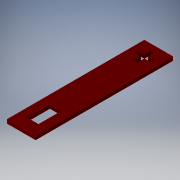
# Autodesk Inventor part: Brazo_Superior
Saved by Autodesk Inventor 2019 (Build 230136000, 136)
## iProperties
Created: 2020-02-09
Part Number: Brazo_Superior
Material: Generic
Document SubType Name: Modeling
Designer: Omar
Density: 1 g/cm^3
Appearance: Default
Author: Omar
Autodesk Inventor part; units mm, degrees
ref_plane "YZ Plane" through (0, 0, 0) normal (1, 0, 0) x (0, 1, 0)
ref_plane "XZ Plane" through (0, 0, 0) normal (0, 1, 0) x (-1, 0, 0)
ref_plane "XY Plane" through (0, 0, 0) normal (0, 0, 1) x (1, 0, 0)
sketch "Sketch1" plane through (0, 0, 0) normal (0, 1, 0) x (-1, 0, 0)
  line L0 (88.91, 20) -> (92.09, 20)
  line L1 (102.5, 9.09) -> (87.5, 9.09)
  line L2 (87.5, 9.09) -> (87.5, 5.91)
  line L3 (87.5, 5.91) -> (102.5, 5.91)
  line L4 (102.5, 5.91) -> (102.5, 9.09)
  line L5 (96.59, 15) -> (93.41, 15)
  line L6 (93.41, 15) -> (93.41, 0)
  line L7 (93.41, 0) -> (96.59, 0)
  line L8 (96.59, 0) -> (96.59, 15)
  line L9 (96.59, 15) -> (93.41, 0) construction
  line L10 (93.41, 15) -> (96.59, 0) construction
  line L11 (-7.5, -85.91) -> (-7.5, -89.09)
  line L12 (1.59, -80) -> (-1.59, -80)
  line L13 (-1.59, -80) -> (-1.59, -95)
  line L14 (-1.59, -95) -> (1.59, -95)
  line L15 (1.59, -95) -> (1.59, -80)
  line L16 (-1.59, -80) -> (1.59, -95) construction
  line L17 (7.5, -85.91) -> (-7.5, -85.91)
  line L18 (-7.5, -89.09) -> (7.5, -89.09)
  line L19 (7.5, -89.09) -> (7.5, -85.91)
  line L20 (1.59, -80) -> (-1.59, -95) construction
  line L21 (-5, 10) -> (5, 10)
  line L22 (5, 10) -> (5, -10)
  line L23 (5, -10) -> (-5, -10)
  line L24 (-5, -10) -> (-5, 10)
  line L25 (-5, 10) -> (5, -10) construction
  line L26 (5, 10) -> (-5, -10) construction
  line L27 (12.5, 20) -> (-12.5, 20)
  line L28 (-12.5, 20) -> (-12.5, -100)
  line L29 (-12.5, -100) -> (12.5, -100)
  line L30 (12.5, -100) -> (12.5, 20)
  point P0 (0, 0)
  point P1 (0, 0)
  point P2 (95, 7.5)
  point P3 (0, -87.5)
  point P4 (0, 0)
  dimension "d8" = 15
  dimension "d9" = 3.18
  dimension "d10" = 3.18
  dimension "d11" = 15
  dimension "d12" = 7.5
  dimension "d13" = 1.59
  dimension "d16" = 15
  dimension "d18" = 3.18
  dimension "d19" = 15
  dimension "d20" = 7.5
  dimension "d21" = 1.59
  dimension "d24" = 10
  dimension "d25" = 20
  dimension "d26" = 25
  dimension "d27" = 120
  dimension "d28" = 20
  dimension "d29" = 12.5
  dimension "d30" = 12.5
  dimension "d31" = 12.5
  dimension "d32" = 3.18
  constraints: 62 end point, 12 parallel, 7 midpoint, 6 horizontal, 6 perpendicular, 1 coincident
  measures "d8" distance of L3.end L2.end
  measures "d9" distance of L2.end L1.end
  measures "d10" distance of L7.end L6.end
  measures "d11" distance of L6.end L5.end
  measures "d12" distance from line of L4 point (95, 7.5)
  measures "d13" distance from line of L3 point (95, 7.5)
  measures "d16" distance of L18.end L11.end
  measures "d18" distance of L14.end L13.end
  measures "d19" distance of L13.end L12.end
  measures "d20" distance from line of L19 point (0, -87.5)
  measures "d21" distance from line of L18 point (0, -87.5)
  measures "d24" distance of L22.end L23.end
  measures "d25" distance of L21.end L22.end
  measures "d26" distance of L29.end L28.end
  measures "d27" distance of L29.end L27.start
  measures "d28" distance from line of L27 point (0, 0)
  measures "d29" distance from line of L30 point (0, 0)
  measures "d30" distance from line of L29 point (0, -87.5)
  measures "d31" distance from line of L28 point (0, -87.5)
  measures "d32" distance of L18.end L17.start
extrude "Extrusion1" add sketch "Sketch1" along normal blind 3.18 contours L30 L29 L28 L27
body "Solid1"
